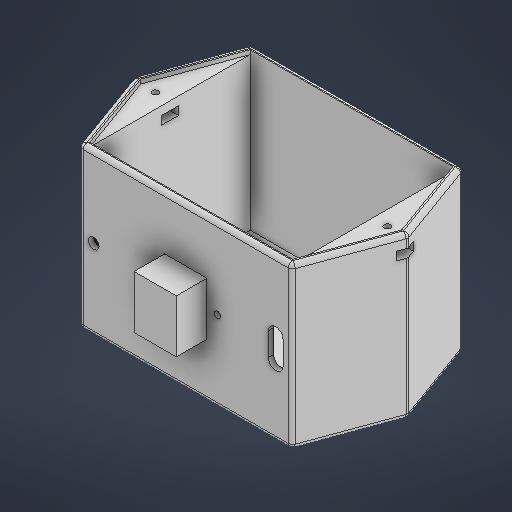
# Autodesk Inventor part: ControllerHead
Saved by Autodesk Inventor 2026.2 (Build 302298010, 298A)
## iProperties
Created: 2026-03-18
Part Number: ControllerHead
Material: Generic
Document SubType Name: Modeling
Designer: barbe
Density: 1 g/cm^3
Appearance: Default
Author: barbe
Autodesk Inventor part; units mm, degrees
ref_plane "YZ Plane" through (0, 0, 0) normal (1, 0, 0) x (0, 1, 0)
ref_plane "XZ Plane" through (0, 0, 0) normal (0, 1, 0) x (-1, 0, 0)
ref_plane "XY Plane" through (0, 0, 0) normal (0, 0, 1) x (1, 0, 0)
sketch "Sketch4" plane through (0, 0, 0) normal (0, 1, 0) x (-1, 0, 0)
  line L0 (50, 40.5) -> (-50, 40.5)
  line L1 (-50, 40.5) -> (-50, -40.5)
  line L2 (-50, -40.5) -> (50, -40.5)
  line L3 (50, -40.5) -> (50, 40.5)
  line L4 (50, 40.5) -> (-50, -40.5) construction
  line L5 (-50, 40.5) -> (50, -40.5) construction
  line L6 (45.72, 36.195) -> (-45.72, 36.195)
  line L7 (-45.72, 36.195) -> (-45.72, -36.195)
  line L8 (-45.72, -36.195) -> (45.72, -36.195)
  line L9 (45.72, -36.195) -> (45.72, 36.195)
  line L10 (45.72, 36.195) -> (-45.72, -36.195) construction
  line L11 (-45.72, 36.195) -> (45.72, -36.195) construction
  line L12 (48, 38) -> (-48, 38)
  line L13 (-48, 38) -> (-48, -38)
  line L14 (-48, -38) -> (48, -38)
  line L15 (48, -38) -> (48, 38)
  line L16 (48, 38) -> (-48, -38) construction
  line L17 (-48, 38) -> (48, -38) construction
  line L18 (-50, 40.5) -> (-64.7408, 0)
  line L19 (-50, 40.5) -> (-6.9008, 40.5) construction
  line L20 (-50, -40.5) -> (-64.7408, 0)
  line L21 (-50, -40.5) -> (-6.9008, -40.5) construction
  line L22 (0, 0) -> (72.39, 0) construction
  line L23 (0, -40.5) -> (0, 40.5)
  line L24 (50, 40.5) -> (64.7408, 0)
  line L25 (50, -40.5) -> (64.7408, 0)
  line L26 (64.7408, 0) -> (-64.7408, 0)
  circle A0 centre (25.4, 19.685) radius 3
  circle A1 centre (10.16, 19.685) radius 3
  circle A2 centre (-25.4, 19.685) radius 3
  circle A3 centre (-10.16, 19.685) radius 3
  circle A4 centre (0, 29.845) radius 3
  circle A5 centre (0, 9.525) radius 3
  line L27 (45.72, -36.195) -> (48.26, -36.195) construction
  line L28 (43.18, -33.655) -> (5.08, -33.655)
  line L29 (5.08, -33.655) -> (5.08, 4.445)
  line L30 (5.08, 4.445) -> (43.18, 4.445)
  line L31 (43.18, 4.445) -> (43.18, -33.655)
  line L32 (5.08, -14.605) -> (24.13, -14.605) construction
  circle A6 centre (24.13, -14.605) radius 14.25
  line L33 (-43.18, -33.655) -> (-5.08, -33.655)
  line L34 (-5.08, -33.655) -> (-5.08, 4.445)
  line L35 (-5.08, 4.445) -> (-43.18, 4.445)
  line L36 (-43.18, 4.445) -> (-43.18, -33.655)
  circle A7 centre (-24.13, -14.605) radius 14.25
  line L37 (-48, -38) -> (-61.8309, 0)
  line L38 (-48, -38) -> (-7.5612, -38) construction
  line L39 (-48, 38) -> (-61.8309, 0)
  line L40 (-48, 38) -> (-7.5612, 38) construction
  line L41 (48, -38) -> (61.8309, 0)
  line L42 (48, 38) -> (61.8309, 0)
  circle A8 centre (54.9155, 0) radius 1.5
  circle A9 centre (-54.9155, 0) radius 1.5
  point P0 (0, 36.195)
  dimension "d52" = 100
  dimension "d53" = 81
  dimension "d54" = 91.44
  dimension "d55" = 72.39
  dimension "d56" = 96
  dimension "d57" = 76
  dimension "d58" = 110
  dimension "d59" = 110
  dimension "d62" = 6
  dimension "d63" = 20.32
  dimension "d64" = 16.51
  dimension "d65" = 6
  dimension "d66" = 15.24
  dimension "d67" = 6
  dimension "d68" = 6.35
  dimension "d69" = 6
  dimension "d70" = 20.32
  dimension "d73" = 38.1
  dimension "d74" = 38.1
  dimension "d75" = 2.54
  dimension "d76" = 2.54
  dimension "d79" = 28.5
  dimension "d83" = 110
  dimension "d84" = 110
  dimension "d86" = 3
  dimension "d112" = 54.9155
  constraints: 86 end point, 12 horizontal, 11 midpoint, 10 centre point, 10 symmetric about line, 8 parallel, 4 equal length, 4 perpendicular, 4 point on line, 1 coincident, 4 other
  measures "d52" distance of L2.end L1.end
  measures "d53" distance of L1.end L0.end
  measures "d54" distance of L8.end L7.end
  measures "d55" distance of L7.end L6.end
  measures "d56" distance of L14.end L13.end
  measures "d57" distance of L13.end L12.end
  measures "d58" angle of L18 L19
  measures "d59" angle of L21 L20
  measures "d62" diameter of A0
  measures "d63" distance from line of L9 A0.centre
  measures "d64" distance from line of L6 A0.centre
  measures "d65" diameter of A1
  measures "d66" distance of A1.centre A0.centre
  measures "d67" diameter of A4
  measures "d68" distance of point (0, 36.195) A4.centre
  measures "d69" diameter of A5
  measures "d70" distance of A4.centre A5.centre
  measures "d73" distance of L29.end L30.end
  measures "d74" distance of L28.end L29.end
  measures "d75" distance between parallel lines of L8 L28
  measures "d76" distance between parallel lines of L9 L31
  measures "d79" diameter of A6
  measures "d83" angle of L38 L37
  measures "d84" angle of L39 L40
  measures "d86" diameter of A8
  measures "d112" distance from line of L23 A8.centre
extrude "Extrusion7" add sketch "Sketch4" along normal blind 76 contours L3 L42 L12 L23 L0 | L24 L26 L42 L3 | L23 L12 L39 L1 L0 | L25 L3 L41 L26 | L1 L39 L26 L18 | L2 L23 L14 L41 L3 | L26 L37 L1 L20 | L2 L1 L37 L14 L23
extrude "Extrusion8" add sketch "Sketch4" along normal blind 74 contours L42 L26 A8 L3 | L3 L26 L15 L42 | L26 A8 L41 L3 | L3 L41 L15 L26 | L39 L13 L26 L1 | L1 L26 A9 L39 | L26 L13 L37 L1 | L1 L37 L26 A9
fillet "Fillet4" radius 2 18 edges at (0, 0, -40.5) (-50, 38, -40.5) (0, 76, -40.5) (50, 38, -40.5) (57.3704, 0, -20.25) (57.3704, 76, -20.25) (64.7408, 38, 0) (57.3704, 0, 20.25) (57.3704, 76, 20.25) (50, 38, 40.5) (-57.3704, 0, 20.25) (-50, 38, 40.5) (-57.3704, 76, 20.25) (-64.7408, 38, 0) (0, 0, 40.5) (-57.3704, 0, -20.25) (0, 76, 40.5) (-57.3704, 76, -20.25)
extrude "Extrusion11" add sketch "Sketch4" along normal blind 70 contours A8 L26 | L26 A8 | A9 L26 | L26 A9
sketch "Sketch5" plane through (-48.5996, 74, 40.5) normal (0, 0, 1) x (1, 0, 0)
  line L0 (0, -72) -> (97.1992, -72) projected
  line L1 (97.1992, -72) -> (0, -72)
  line L2 (97.1992, 0) -> (0, 0) projected
  line L3 (0, -72) -> (0, 0)
  line L4 (0, 0) -> (97.1992, 0)
  line L5 (97.1992, 0) -> (97.1992, -72)
  line L6 (97.1992, -36) -> (0, -36)
  line L7 (48.5996, -72) -> (48.5996, 0)
  line L8 (58.5996, -23.5) -> (38.5996, -23.5)
  line L9 (38.5996, -23.5) -> (38.5996, -48.5)
  line L10 (38.5996, -48.5) -> (58.5996, -48.5)
  line L11 (58.5996, -48.5) -> (58.5996, -23.5)
  line L12 (58.5996, -23.5) -> (38.5996, -48.5) construction
  line L13 (38.5996, -23.5) -> (58.5996, -48.5) construction
  circle A0 centre (33.5996, -36) radius 1.5
  circle A1 centre (63.5996, -36) radius 1.5
  line L14 (67.8423, -21) -> (29.3569, -21)
  line L15 (29.3569, -21) -> (29.3569, -51)
  line L16 (29.3569, -51) -> (67.8423, -51)
  line L17 (67.8423, -51) -> (67.8423, -21)
  line L18 (67.8423, -21) -> (29.3569, -51) construction
  line L19 (29.3569, -21) -> (67.8423, -51) construction
  line L20 (91.1992, -30.5) -> (91.1992, -41.5) construction
  line L21 (87.6992, -30.5) -> (87.6992, -41.5)
  line L22 (94.6992, -41.5) -> (94.6992, -30.5)
  arc A2 (94.6992, -30.5) -> (87.6992, -30.5) centre (91.1992, -30.5) ccw
  arc A3 (87.6992, -41.5) -> (94.6992, -41.5) centre (91.1992, -41.5) ccw
  line L23 (97.1992, 0) -> (97.1992, -72) projected
  circle A4 centre (5, -36) radius 2.5
  line L24 (0, -72) -> (0, 0) projected
  point P0 (48.5996, -74)
  point P1 (48.5996, -36)
  point P2 (91.1992, -36)
  dimension "d115" = 20
  dimension "d118" = 3
  dimension "d119" = 15
  dimension "d134" = 25
  dimension "d135" = 30
  dimension "d176" = 5.5
  dimension "d177" = 7
  dimension "d178" = 6
  dimension "d179" = 5
  dimension "d180" = 5
  constraints: 44 end point, 12 midpoint, 7 equal length, 5 centre point, 5 perpendicular, 4 point on circle, 4 tangent, 3 point on line, 2 horizontal, 1 symmetric about line, 1 other
  measures "d115" distance of L10.end L9.end
  measures "d118" diameter of A0
  measures "d119" distance from line of L7 A0.centre
  measures "d134" distance of L8.start L10.end
  measures "d135" distance of L15.end L14.end
  measures "d176" distance of point (91.199, -36) L20.end
  measures "d177" diameter of A3
  measures "d178" distance of point (91.199, -36) point (97.199, -36)
  measures "d179" diameter of A4
  measures "d180" distance of point (0, -36) A4.centre
extrude "Extrusion12" add sketch "Sketch5" along normal blind 14.5 contours L10 L9 L6 L7 | L7 L6 L11 L10 | L7 L8 L11 L6 | L6 L9 L8 L7
extrude "Extrusion14" cut sketch "Sketch5" along normal blind 10 and the other way blind 5 contours A0 L6 | L6 A0 | A1 L6 | L6 A1
extrude "Extrusion15" add sketch "Sketch4" along normal blind 2 contours L23 L6 L7 L26 L13 L12 | L12 L15 L26 L9 L6 L23 | L23 A4 A5 L26 L34 L35 L36 L7 L6 | L6 L9 L26 L31 L30 L29 L23 A5 A4 | L15 L14 L23 L8 L9 L26 | L26 L7 L8 L23 L14 L13 | L9 L8 L23 L26 L29 L28 L31 | L26 L36 L33 L34 L23 L8 L7 | L31 L28 L29 L26 | L26 L29 L30 L31 | L36 L35 L34 L26 | L26 L34 L33 L36
chamfer "Chamfer10" distance 1.5 angle 45 2 edges at (38.38, 0, -14.605) (-9.88, 0, -14.605)
chamfer "Chamfer11" distance 0.5 angle 45 6 edges at (28.4, 0, 19.685) (13.16, 0, 19.685) (3, 0, 9.525) (-7.16, 0, 19.685) (3, 0, 29.845) (-22.4, 0, 19.685)
extrude "Extrusion16" cut sketch "Sketch5" against normal up to surface (2.5 mm away) contours A4 L6 | L6 A4 | L22 A3 L21 L6 | L6 L21 A2 L22
sketch "Sketch6" plane through (-48, 74, 38) normal (1, 0, 0) x (0, 0, -1)
  line L0 (38, -4) -> (42, -4)
  line L1 (42, -4) -> (42, -8)
  line L2 (42, -8) -> (38, -8)
  line L3 (38, -8) -> (38, -4)
  line L4 (38, -4) -> (38, -8)
  line L5 (38, -8) -> (34, -8)
  line L6 (34, -8) -> (34, -4)
  line L7 (34, -4) -> (38, -4)
  line L8 (0, 0) -> (76, 0) projected
  point P0 (38, -74)
  point P1 (38, 0)
  dimension "d183" = 4
  dimension "d184" = 4
  dimension "d185" = 4
  dimension "d186" = 4
  constraints: 16 end point, 4 parallel, 3 perpendicular, 1 horizontal, 1 midpoint
  measures "d183" distance of L0.start L0.end
  measures "d184" distance of L0.end L1.end
  measures "d185" distance of L2.end L5.end
  measures "d186" distance of point (38, 0) L0.start
extrude "Extrusion17" cut sketch "Sketch6" along normal through all both and the other way through all
body "Solid3"
